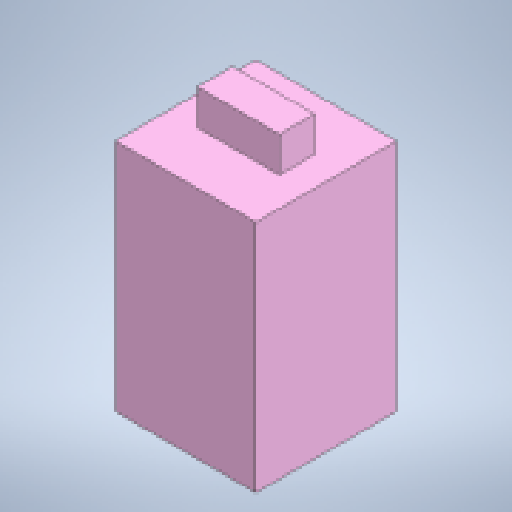
# Autodesk Inventor part: Soda barrel
Saved by Autodesk Inventor 2025.4 (Build 294407000, 407)
## iProperties
Created: 2025-03-29
Part Number: Soda barrel
Material: Generic
Document SubType Name: Modeling
Designer: pokla
Density: 1 g/cm^3
Appearance: Default
Author: pokla
Autodesk Inventor part; units mm, degrees
ref_plane "YZ Plane" through (0, 0, 0) normal (1, 0, 0) x (0, 1, 0)
ref_plane "XZ Plane" through (0, 0, 0) normal (0, 1, 0) x (-1, 0, 0)
ref_plane "XY Plane" through (0, 0, 0) normal (0, 0, 1) x (1, 0, 0)
sketch "Sketch1" plane through (0, 0, 0) normal (0, 0, 1) x (1, 0, 0)
  line L0 (-300, 300) -> (300, 300)
  line L1 (300, 300) -> (300, -300)
  line L2 (300, -300) -> (-300, -300)
  line L3 (-300, -300) -> (-300, 300)
  line L4 (-300, -300) -> (300, 300) construction
  point P0 (0, 0)
  point P1 (0, 0)
  dimension "d0" = 600
  dimension "d1" = 600
  constraints: 10 end point, 2 parallel, 1 coincident, 1 horizontal, 1 midpoint, 1 perpendicular
  measures "d0" distance of L0.start L0.end
  measures "d1" distance between parallel lines of L2 L0
extrude "Extrusion1" add sketch "Sketch1" along normal blind 1000
sketch "Sketch2" plane through (0, 0, 1000) normal (0, 0, 1) x (1, 0, 0)
  line L0 (-175, 75) -> (175, 75)
  line L1 (175, 75) -> (175, -75)
  line L2 (175, -75) -> (-175, -75)
  line L3 (-175, -75) -> (-175, 75)
  line L4 (-175, 75) -> (175, -75) construction
  line L5 (175, 75) -> (-175, -75) construction
  point P0 (0, 0)
  dimension "d4" = 350
  dimension "d5" = 150
  constraints: 12 end point, 2 midpoint, 2 parallel, 1 horizontal, 1 perpendicular
  measures "d4" distance of L1.end L2.end
  measures "d5" distance of L0.end L1.end
extrude "Extrusion2" add sketch "Sketch2" along normal blind 150
equation "\"d0\" = Длина"
equation "\"d1\" = Ширина"
equation "\"d2\" = Высота"
equation "\"Длина\" = 600"
equation "\"Ширина\" = 600"
equation "\"Высота\" = 1000"
body "Solid1"
